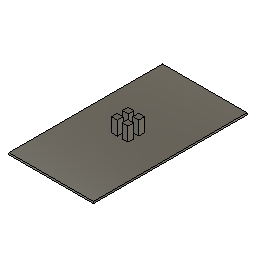
updatedkey v3 (Autodesk Fusion 360 design; units mm, degrees)
Autodesk Fusion 360 part; units mm, degrees
note: some values were not read from the file. Chosen so that the rebuilt part matches the saved one: which bodies a step acts on.
sketch "Sketch1" plane through (0, 0, 0) normal (0, 0, 1) x (1, 0, 0)
  line L0 (2.15, 0.675) -> (-2.15, 0.675)
  line L1 (-2.15, 0.675) -> (-2.15, -0.675)
  line L2 (-2.15, -0.675) -> (2.15, -0.675)
  line L3 (2.15, -0.675) -> (2.15, 0.675)
  line L4 (2.15, 0.675) -> (-2.15, -0.675) construction
  line L5 (-2.15, 0.675) -> (2.15, -0.675) construction
  line L6 (0.6, 2.15) -> (-0.6, 2.15)
  line L7 (-0.6, 2.15) -> (-0.6, -2.15)
  line L8 (-0.6, -2.15) -> (0.6, -2.15)
  line L9 (0.6, -2.15) -> (0.6, 2.15)
  line L10 (0.6, 2.15) -> (-0.6, -2.15) construction
  line L11 (-0.6, 2.15) -> (0.6, -2.15) construction
  line L12 (2.15, 2.15) -> (-2.15, 2.15)
  line L13 (-2.15, 2.15) -> (-2.15, -2.15)
  line L14 (-2.15, -2.15) -> (2.15, -2.15)
  line L15 (2.15, -2.15) -> (2.15, 2.15)
  line L16 (2.15, 2.15) -> (-2.15, -2.15) construction
  line L17 (-2.15, 2.15) -> (2.15, -2.15) construction
  dimension "d1" = 4.3
  dimension "d2" = 1.35
  dimension "d3" = 1.2
  dimension "d4" = 4.3
  dimension "d5" = 4.3
  dimension "d6" = 4.3
  constraint horizontal L0
  constraint perpendicular L0 L1
  constraint parallel L0 L2
  constraint parallel L1 L3
  constraint coincident L4 origin
  constraint coincident L5 origin
  constraint horizontal L6
  constraint perpendicular L6 L7
  constraint parallel L6 L8
  constraint parallel L7 L9
  constraint coincident L10 origin
  constraint coincident L11 origin
  constraint horizontal L12
  constraint perpendicular L12 L13
  constraint parallel L12 L14
  constraint parallel L13 L15
  constraint coincident L16 origin
  constraint coincident L17 origin
  measures "d1" distance of L1.end L2.end
  measures "d2" distance of L0.end L1.end
  measures "d3" distance of L7.end L8.end
  measures "d4" distance of L6.end L7.end
  measures "d5" distance of L13.end L14.end
  measures "d6" distance of L12.end L13.end
extrude "Extrude1" add sketch "Sketch1" along normal blind 3.6 contours L0 L9 L12 L15 | L2 L9 L14 L15 | L0 L7 L12 L13 | L2 L7 L13 L14 makes body 1 at (-1.6333, -2.15, 1.2) makes body 2 at (-1.1167, 2.15, 1.2) makes body 3 at (1.1167, -2.15, 1.2) makes body 4 at (1.6333, 0.675, 1.2)
sketch "Sketch2" plane through (0, 0, 0) normal (0, 0, 1) x (1, 0, 0)
  line L0 (11, 20) -> (-11, 20)
  line L1 (-11, 20) -> (-11, -20)
  line L2 (-11, -20) -> (11, -20)
  line L3 (11, -20) -> (11, 20)
  line L4 (11, 20) -> (-11, -20) construction
  line L5 (-11, 20) -> (11, -20) construction
  dimension "d9" = 22
  dimension "d10" = 40
  constraint horizontal L0
  constraint perpendicular L0 L1
  constraint parallel L0 L2
  constraint parallel L1 L3
  constraint coincident L4 origin
  constraint coincident L5 origin
  measures "d9" distance of L1.end L2.end
  measures "d10" distance of L0.end L1.end
extrude "Extrude2" add sketch "Sketch2" against normal blind 1.5 bodies 1
chamfer "Chamfer1" distance 1 angle 45 4 edges at (-11, 0, -1.5) (0, -20, -1.5) (11, 0, -1.5) (0, 20, -1.5) on bodies 1
